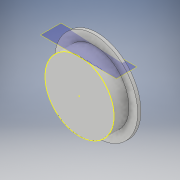
# Autodesk Inventor part: coilpiece2
Saved by Autodesk Inventor 2018 (Build 220112000, 112)
## iProperties
Created: 2019-04-09
Part Number: coilpiece2
Material: Generic
Document SubType Name: Modeling
Designer: F8PLTW
Density: 1 g/cm^3
Appearance: Default
Author: F8PLTW
Autodesk Inventor part; units mm, degrees
ref_plane "YZ Plane" through (0, 0, 0) normal (1, 0, 0) x (0, 1, 0)
ref_plane "XZ Plane" through (0, 0, 0) normal (0, 1, 0) x (-1, 0, 0)
ref_plane "XY Plane" through (0, 0, 0) normal (0, 0, 1) x (1, 0, 0)
sketch "Sketch1" plane through (0, 0, 0) normal (0, 0, 1) x (1, 0, 0)
  circle A0 centre (0, 0) radius 28.194
  dimension "d0" = 56.388
  constraints: 1 centre point, 1 coincident
  measures "d0" diameter of A0
extrude "Extrusion1" add sketch "Sketch1" along normal blind 15.24
sketch "Sketch2" plane through (0, 0, 15.24) normal (0, 0, 1) x (1, 0, 0)
  circle A0 centre (0, 0) radius 28.194 projected
  line L0 (0, 28.194) -> (19.1738, 28.194) construction
  constraints: 2 end point, 2 horizontal, 1 vertical alignment, 1 other
ref_plane "Work Plane1" through (0, 28.194, 15.24) normal (0, -1, 0) x (1, 0, 0)
sketch "Sketch3" plane through (0, 28.194, 15.24) normal (0, -1, 0) x (1, 0, 0)
  line L0 (-28.194, -15.24) -> (28.194, -15.24) projected
  line L1 (-28.194, -15.24) -> (37.5113, -11.7965)
  line L2 (-28.194, -15.24) -> (37.6014, -15.24) construction
  line L3 (37.5113, -11.7965) -> (37.5113, -25.6929)
  line L4 (37.5113, -25.6929) -> (-28.194, -15.24)
  point P0 (0, -15.24)
  dimension "d3" = 3
  constraints: 8 end point, 1 equal length, 1 horizontal, 1 perpendicular
  measures "d3" angle of L2 L1
extrude "Extrusion2" cut sketch "Sketch3" along normal blind 152.4
sketch "Sketch4" plane through (0, 0, 1.4776) normal (0.052336, 0, -0.9986295) x (-0.9986295, 0, -0.052336)
  circle A0 centre (0.0773, 0) radius 35.814
  dimension "d6" = 71.628
  constraints: 1 centre point, 1 coincident
  measures "d6" diameter of A0
extrude "Extrusion3" add sketch "Sketch4" along normal blind 2.54
body "Solid1"
